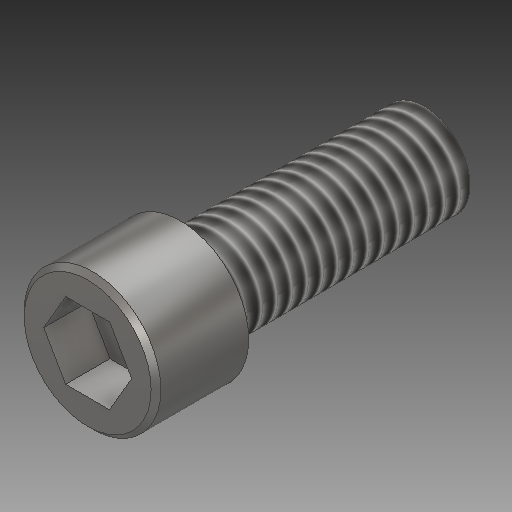
# Autodesk Inventor part: 3-8-16 UNC Bolt
Saved by Autodesk Inventor 2018 (Build 220112000, 112)
## iProperties
Created: 2018-01-08
Part Number: 3-8-16 UNC Bolt
Material: Stainless Steel
Document SubType Name: Modeling
Designer: 232963
Density: 8 g/cm^3
Appearance: Semi-Polished
Mass: 24.6926 g
Surface Area: 16.2245 cm^2
Volume: 3.08658 cm^3
Author: 232963
Autodesk Inventor part; units mm, degrees
ref_plane "YZ Plane" through (0, 0, 0) normal (1, 0, 0) x (0, 1, 0)
ref_plane "XZ Plane" through (0, 0, 0) normal (0, 1, 0) x (-1, 0, 0)
ref_plane "XY Plane" through (0, 0, 0) normal (0, 0, 1) x (1, 0, 0)
sketch "Sketch1" plane through (0, 0, 0) normal (0, 0, 1) x (1, 0, 0)
  circle A0 centre (0, 0) radius 7.112
  dimension "d0" = 14.224
  constraints: 1 centre point, 1 coincident
  measures "d0" diameter of A0
extrude "Extrusion1" add sketch "Sketch1" along normal blind 9.652
sketch "Sketch2" plane through (0, 0, 9.652) normal (0, 0, 1) x (1, 0, 0)
  line L0 (2.2997, 3.9555) -> (4.5754, -0.0139)
  line L1 (4.5754, -0.0139) -> (2.2757, -3.9693)
  line L2 (2.2757, -3.9693) -> (-2.2997, -3.9555)
  line L3 (-2.2997, -3.9555) -> (-4.5754, 0.0139)
  line L4 (-4.5754, 0.0139) -> (-2.2757, 3.9693)
  line L5 (-2.2757, 3.9693) -> (2.2997, 3.9555)
  point P0 (0, 0)
  point P1 (0, 0)
  dimension "d3" = 7.9248
  constraints: 12 end point, 1 coincident, 13 other
  measures "d3" distance between parallel lines of L2 L5
extrude "Extrusion2" cut sketch "Sketch2" against normal blind 4.6228
chamfer "Chamfer1" distance 0.508 angle 45 1 edges at (-7.112, 0, 9.652)
sketch "Sketch3" plane through (0, 0, 0) normal (0, 0, -1) x (-1, 0, 0)
  circle A0 centre (0, 0) radius 4.7625
  dimension "d9" = 9.525
  constraints: 1 centre point, 1 coincident
  measures "d9" diameter of A0
extrude "Extrusion3" add sketch "Sketch3" along normal blind 25.4
thread "Thread1" size "3/8-16 UNC" class "2A" standard "ANSI Unified Screw Threads" full length
body "Solid1"
